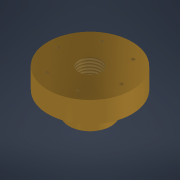
# Autodesk Inventor part: Tuerca
Saved by Autodesk Inventor 2022 (Build 260153000, 153)
## iProperties
Created: 2021-09-10
Part Number: Tuerca
Material: Steel, Mild, Welded
Document SubType Name: Modeling
Designer: Andres
Density: 7.85 g/cm^3
Appearance: Brass - Satin
Author: Andres
Autodesk Inventor part; units mm, degrees
ref_plane "YZ Plane" through (0, 0, 0) normal (1, 0, 0) x (0, 1, 0)
ref_plane "XZ Plane" through (0, 0, 0) normal (0, 1, 0) x (-1, 0, 0)
ref_plane "XY Plane" through (0, 0, 0) normal (0, 0, 1) x (1, 0, 0)
sketch "Sketch1" plane through (0, 0, 0) normal (0, 1, 0) x (-1, 0, 0)
  circle A0 centre (0, 0) radius 8
  circle A1 centre (0, 0) radius 15
  dimension "d0" = 16
  dimension "d1" = 30
  constraints: 2 centre point, 2 coincident
  measures "d0" diameter of A0
  measures "d1" diameter of A1
extrude "Extrusion1" add sketch "Sketch1" along normal mid plane 30
thread "Thread1" size "TR16x2" class "7H" standard "ISO Metric Trapezoidal Threads" full length
sketch "Sketch2" plane through (0, 15, 0) normal (0, -1, 0) x (1, 0, 0)
  circle A0 centre (0, 0) radius 30
  circle A1 centre (0, 0) radius 15 projected
  circle A2 centre (0, 0) radius 8 projected
  dimension "d6" = 60
  constraints: 1 centre point, 1 coincident
  measures "d6" diameter of A0
extrude "Extrusion2" add sketch "Sketch2" along normal blind 15 contours A0
sketch "Sketch4" plane through (0, 0, 0) normal (0, -1, 0) x (-1, 0, 0)
  circle A0 centre (0, 0) radius 30 projected
  circle A1 centre (0, 0) radius 8 projected
  circle A2 centre (0, 0) radius 15
  circle A3 centre (0, 0) radius 23.5
  dimension "d11" = 30
  dimension "d15" = 47
  constraints: 2 centre point, 2 coincident
  measures "d11" diameter of A2
  measures "d15" diameter of A3
extrude "Extrusion3" cut sketch "Sketch4" against normal blind 4 contours A3
sketch "Sketch5" plane through (0, 15, 0) normal (0, -1, 0) x (-1, 0, 0)
  circle A0 centre (0, 0) radius 22.5 construction
  point P0 (22.5, 0)
  dimension "diam_hole_tuerca" = 45
  constraints: 2 horizontal alignment, 1 coincident, 2 other
hole "Hole1" at (-22.5, 15, 0) direction (0, -1, 0) diameter 2.459 depth 8.8 tip angle 118 thread size "M3x0.5" class "6H" standard "ISO Metric profile"
pattern_circular "Circular Pattern1" count 6 over 360 about axis through (0, 0, 0) along (0, 1, 0) of "Hole1"
body "Solid1"
